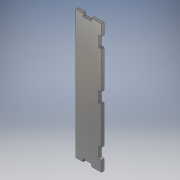
# Autodesk Inventor part: 1-8inch_Top1_1-Part
Saved by Autodesk Inventor 2018 (Build 220112000, 112)
## iProperties
Created: 2018-02-01
Part Number: 1-8inch_Top1_1-Part
Material: Generic
Document SubType Name: Modeling
Designer: Angie
Density: 1 g/cm^3
Appearance: Default
Author: Angie
Autodesk Inventor part; units mm, degrees
ref_plane "YZ Plane" through (0, 0, 0) normal (1, 0, 0) x (0, 1, 0)
ref_plane "XZ Plane" through (0, 0, 0) normal (0, 1, 0) x (-1, 0, 0)
ref_plane "XY Plane" through (0, 0, 0) normal (0, 0, 1) x (1, 0, 0)
sketch "Sketch1" plane through (0, 0, 0) normal (0, 0, 1) x (1, 0, 0)
  line L0 (-21.5, -147.1375) -> (-21.5, -148.5)
  line L1 (-30, -148.5) -> (-30, 0.5)
  line L2 (-30, 0.5) -> (-21.5, 0.5)
  line L3 (-21.5, 0.5) -> (-21.5, -2.675)
  line L4 (-11.5, -2.5) -> (-11.5, 0.5)
  line L5 (-11.5, 0.5) -> (0, 0.5)
  line L6 (0, 0.5) -> (0, -12.2)
  line L7 (0, -29) -> (0, -68.5562)
  line L8 (0, -81.2562) -> (0, -119)
  line L9 (0, -137.6125) -> (0, -148.5)
  line L10 (-11.5, -148.5) -> (-11.5, -147.1375)
  line L11 (-21.5, -147.1375) -> (-21.5, -148.5)
  line L12 (-30, -148.5) -> (-30, 0.5)
  line L13 (-30, 0.5) -> (-21.5, 0.5)
  line L14 (-21.5, 0.5) -> (-21.5, -2.675)
  line L15 (-11.5, -2.5) -> (-11.5, 0.5)
  line L16 (-11.5, 0.5) -> (0, 0.5)
  line L17 (0, 0.5) -> (0, -12.2)
  line L18 (0, -29) -> (0, -68.5562)
  line L19 (0, -81.2562) -> (0, -119)
  line L20 (0, -137.6125) -> (0, -148.5)
  line L21 (-11.5, -148.5) -> (-11.5, -147.1375)
  line L22 (-30, -150.3125) -> (-30, 0.5)
  line L23 (-11.5, -147.1375) -> (-11.5, -150.3125)
  line L24 (-21.5, -150.3125) -> (-21.5, -147.1375)
  line L25 (-11.5, -150.3125) -> (0, -150.3125)
  line L26 (0, -150.3125) -> (0, -147.1375)
  line L27 (-11.5, -147.1375) -> (-21.5, -147.1375)
  line L28 (-30, -147.1375) -> (-30, -150.3125)
  line L29 (0, -150.3125) -> (-11.5, -150.3125)
  line L30 (-21.5, -150.3125) -> (-30, -150.3125)
  line L31 (-30, 0.5) -> (-21.5, 0.5)
  line L32 (-11.5, 0.5) -> (0, 0.5)
  line L33 (0, 0.5) -> (0, -2.675)
  line L34 (-11.5, -2.675) -> (-21.5, -2.675)
  line L35 (-30, -2.675) -> (-30, 0.5)
  line L36 (-11.5, 0.5) -> (-11.5, -2.675)
  line L37 (-11.5, -2.675) -> (-21.5, -2.675)
  line L38 (-21.5, -2.675) -> (-21.5, 0.5)
  line L39 (-30, 0.5) -> (-21.5, 0.5)
  line L40 (-11.5, 0.5) -> (0, 0.5)
  line L41 (0, 0.5) -> (-3.175, 0.5)
  line L42 (-3.175, -150.3125) -> (0, -150.3125)
  line L43 (-3.175, 0.5) -> (0, 0.5)
  line L44 (0, 0.5) -> (0, -12.2)
  line L45 (0, -12.2) -> (-3.175, -12.2)
  line L46 (-3.175, -12.2) -> (0, -12.2)
  line L47 (0, -24.9) -> (-3.175, -24.9)
  line L48 (-3.175, -24.9) -> (-3.175, -12.2)
  line L49 (-3.175, -24.9) -> (0, -24.9)
  line L50 (0, -24.9) -> (0, -68.5562)
  line L51 (0, -68.5562) -> (-3.175, -68.5562)
  line L52 (-3.175, -68.5562) -> (0, -68.5562)
  line L53 (0, -81.2562) -> (-3.175, -81.2562)
  line L54 (-3.175, -81.2562) -> (-3.175, -68.5562)
  line L55 (-3.175, -81.2562) -> (0, -81.2562)
  line L56 (0, -81.2562) -> (0, -124.9125)
  line L57 (0, -124.9125) -> (-3.175, -124.9125)
  line L58 (-3.175, -124.9125) -> (0, -124.9125)
  line L59 (0, -137.6125) -> (-3.175, -137.6125)
  line L60 (-3.175, -137.6125) -> (-3.175, -124.9125)
  line L61 (-3.175, -150.3125) -> (0, -150.3125)
  line L62 (0, -150.3125) -> (0, -137.6125)
  line L63 (0, -137.6125) -> (-3.175, -137.6125)
  line L64 (0, -137.6125) -> (0, -150.3125)
  line L65 (0, -150.3125) -> (0, -137.6125)
  line L66 (0, -124.9125) -> (0, -81.2562)
  line L67 (0, -81.2562) -> (0, -124.9125)
  line L68 (0, -68.5562) -> (0, -24.9)
  line L69 (0, -12.2) -> (0, 0.5)
  line L70 (0, 0.5) -> (0, -12.2)
  line L71 (0, -24.9) -> (0, -68.5562)
  line L72 (-3.175, -12.2) -> (-3.175, -24.9)
  line L73 (-3.175, -68.5562) -> (-3.175, -81.2562)
  line L74 (-3.175, -124.9125) -> (-3.175, -137.6125)
  point P0 (0, 0)
  constraints: 150 end point, 35 parallel, 18 perpendicular, 13 horizontal, 8 point on line
extrude "Extrusion1" add sketch "Sketch1" along normal blind 3.175
body "Solid1"
